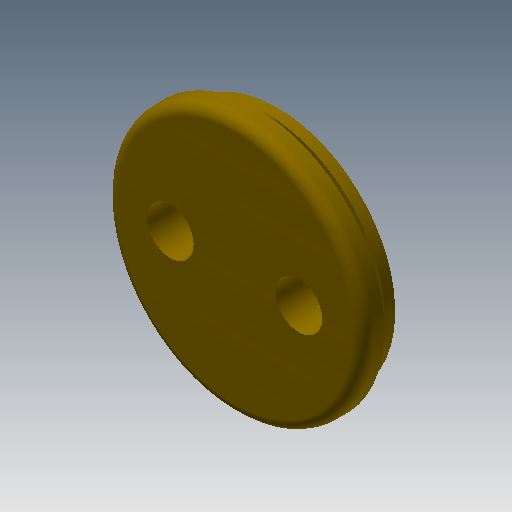
# Autodesk Inventor part: INSULATION-GASKET-2
Saved by Autodesk Inventor 2020 (Build 240152000, 152)
## iProperties
Part Number: INSULATION-GASKET-2
Document SubType Name: Modeling
Created: 2003-04-24
Designer: bakerm
Material: Phenolic
Density: 1.38 g/cm^3
Appearance: Gold
Description: Enclosure Unit Insulation
Mass: 64.6588 g
Surface Area: 134.73 cm^2
Volume: 46.8542 cm^3
Control State: 0
Master: False
Checked Out: False
Last Check In By: bakerm
Last Check In Date: 2003-05-23
Shininess: 64.0
Length Units: 11272
Angle Units: 11279
Time Units: 11290
Mass Units: 11286
Length Display Precision: 3
Angle Display Precision: 2
Compacted: True
Density: 0.0
Volumn: 0.0
Area: 0.0
PropertySet Name: Model Information
Author: bakerm
Revision Number: A
Autodesk Inventor part; units mm, degrees
ref_plane "YZ Plane" through (0, 0, 0) normal (1, 0, 0) x (0, 1, 0)
ref_plane "XZ Plane" through (0, 0, 0) normal (0, 1, 0) x (-1, 0, 0)
ref_plane "XY Plane" through (0, 0, 0) normal (0, 0, 1) x (1, 0, 0)
sketch "Sketch1" plane through (0, 0, 0) normal (0, 0, 1) x (1, 0, 0)
  circle A0 centre (-78.0974, 78.0974) radius 31.75 projected
  circle A1 centre (-78.0974, 78.0974) radius 38.1
  dimension "d0" = 76.2
  constraints: 1 centre point, 1 coincident, 1 concentric
  measures "d0" diameter of A1
extrude "Extrusion1" add sketch "Sketch1" along normal blind 6.35 contours A0 | A1
extrude "Extrusion2" add sketch "Sketch1" against normal blind 3.175 contours A0
sketch "Sketch3" plane through (-78.0974, 78.0974, -3.175) normal (0, 0, -1) x (-1, 0, 0)
  circle A0 centre (0, 0) radius 31.75 projected
  circle A1 centre (0, 0) radius 34.925
  dimension "d5" = 69.85
  constraints: 1 centre point, 1 coincident, 1 concentric
  measures "d5" diameter of A1
extrude "Extrusion3" add sketch "Sketch3" along normal blind 3.175 contours A0 | A1
fillet "Fillet1" radius 3.175 1 edges at (-116.1974, 78.0974, 6.35)
sketch "Sketch4" plane through (-78.0974, 78.0974, 6.35) normal (0, 0, 1) x (1, 0, 0)
  circle A0 centre (0, 0) radius 34.925 projected
  circle A1 centre (-19.05, 0) radius 6.9166
  circle A2 centre (19.05, 0) radius 6.9166
  dimension "d12" = 19.05
  dimension "d13" = 38.1
  constraints: 2 centre point
  measures "d12" distance of A1.centre A0.centre
  measures "d13" distance of A2.centre A1.centre
extrude "Extrusion4" cut sketch "Sketch4" against normal through all contours A1 | A2
equation "\"d13\" = 2 * d12"
body "Solid1"
